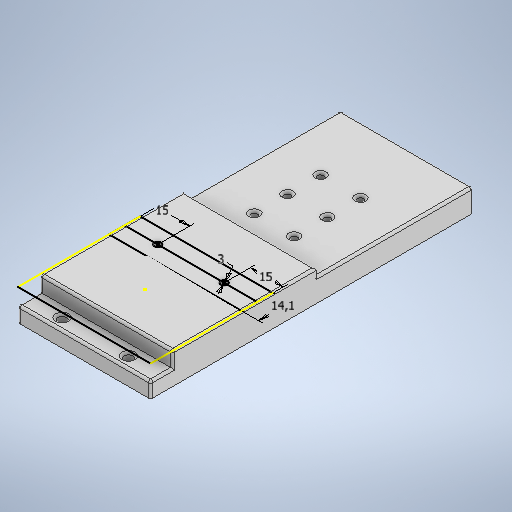
# Autodesk Inventor part: cadre
Saved by Autodesk Inventor 2025.1 (Build 291241000, 241)
## iProperties
Created: 2025-05-14
Part Number: cadre
Material: Générique
Document SubType Name: Modeling
Designer: chapuzet
Density: 1 g/cm^3
Appearance: Par défaut
Author: chapuzet
Autodesk Inventor part; units mm, degrees
ref_plane "YZ Plane" through (0, 0, 0) normal (1, 0, 0) x (0, 1, 0)
ref_plane "XZ Plane" through (0, 0, 0) normal (0, 1, 0) x (-1, 0, 0)
ref_plane "XY Plane" through (0, 0, 0) normal (0, 0, 1) x (1, 0, 0)
sketch "Esquisse1" plane through (0, 0, 0) normal (0, 1, 0) x (-1, 0, 0)
  line L0 (-30, 27.65) -> (30, 27.65)
  line L1 (30, 27.65) -> (30, -27.65)
  line L2 (30, -27.65) -> (-30, -27.65)
  line L3 (-30, -27.65) -> (-30, 27.65)
  line L4 (-30, 27.65) -> (30, -27.65) construction
  line L5 (30, 27.65) -> (-30, -27.65) construction
  point P0 (0, 0)
  dimension "d0" = 60
  dimension "d10" = 55.3
  constraints: 12 end point, 2 midpoint, 2 parallel, 1 horizontal, 1 perpendicular
  measures "d0" distance of L1.end L2.end
  measures "d10" distance of L0.end L1.end
extrude "Extrusion1" add sketch "Esquisse1" along normal blind 14
sketch "Esquisse2" plane through (0, 14, 0) normal (0, 1, 0) x (1, 0, 0)
  line L0 (30, -27.65) -> (30, 27.65) projected
  line L1 (-30, -27.65) -> (30, -27.65)
  line L2 (-30, 27.65) -> (-30, -27.65) projected
  line L3 (-30, 27.65) -> (30, 27.65)
  line L4 (30, 27.65) -> (30, 13.55)
  line L5 (30, 13.55) -> (-30, 13.55)
  line L6 (-30, 13.55) -> (-30, 27.65)
  line L7 (-30, 20.6) -> (30, 20.6)
  circle A0 centre (-15, 20.6) radius 1.5
  circle A1 centre (15, 20.6) radius 1.5
  point P0 (0, 0)
  point P1 (-30, 13.55)
  dimension "d29" = 14.1
  dimension "d40" = 15
  dimension "d41" = 15
  dimension "d42" = 3
  constraints: 12 end point, 3 point on line, 2 centre point, 2 horizontal, 2 midpoint, 2 parallel, 1 equal radius, 1 perpendicular
  measures "d29" distance between parallel lines of L3 L5
  measures "d40" distance from line of L0 A1.centre
  measures "d41" distance from line of L2 A0.centre
  measures "d42" diameter of A1
extrude "Extrusion2" [suppressed]
sketch "Esquisse5" plane through (30, 0, -27.65) normal (0, 0, -1) x (-1, 0, 0)
  line L0 (60, 0) -> (0, 0)
  line L1 (0, 0) -> (0, 14)
  line L2 (0, 14) -> (60, 14)
  line L3 (60, 14) -> (60, 0)
  point P0 (30, 0)
  constraints: 8 end point, 2 parallel, 1 horizontal, 1 perpendicular
extrude "Extrusion4" add sketch "Esquisse5" along normal blind 19.6
sketch "Esquisse6" plane through (30, 0, -47.25) normal (0, 0, -1) x (-1, 0, 0)
  line L0 (0, 0) -> (60, 0) projected
  line L1 (0, 14) -> (0, 0) projected
  line L2 (60, 0) -> (0, 0)
  line L3 (0, 0) -> (0, 10.4)
  line L4 (0, 10.4) -> (60, 10.4)
  line L5 (60, 10.4) -> (60, 0)
  point P0 (30, 0)
  point P1 (0, 15)
  dimension "d17" = 10.4
  constraints: 8 end point, 2 parallel, 1 horizontal, 1 perpendicular, 1 point on line
  measures "d17" distance between parallel lines of L0 L4
extrude "Extrusion5" add sketch "Esquisse6" along normal blind 71
sketch "Esquisse7" plane through (-30, 10.4, -47.25) normal (0, 1, 0) x (1, 0, 0)
  line L0 (0, -74.9) -> (0, 0) projected
  line L1 (0, 71) -> (60, 71) projected
  line L2 (0, 0) -> (60, 0)
  line L3 (60, 0) -> (60, 71)
  line L4 (60, 71) -> (0, 71)
  line L5 (0, 71) -> (0, 0)
  line L6 (21, 11) -> (39, 11)
  line L7 (39, 11) -> (39, 41)
  line L8 (39, 41) -> (21, 41)
  line L9 (21, 41) -> (21, 11)
  line L10 (21, 11) -> (39, 41) construction
  line L11 (39, 11) -> (21, 41) construction
  line L12 (30, 71) -> (30, 0)
  line L13 (39, 26) -> (21, 26)
  circle A0 centre (39, 11) radius 1.5
  circle A1 centre (21, 11) radius 1.5
  circle A2 centre (21, 26) radius 1.5
  circle A3 centre (39, 26) radius 1.5
  circle A4 centre (39, 41) radius 1.5
  circle A5 centre (21, 41) radius 1.5
  point P0 (30, -47.25)
  point P1 (0, -19.6)
  point P2 (30, 26)
  dimension "d20" = 18
  dimension "d21" = 11
  dimension "d22" = 30
  dimension "d23" = 3
  constraints: 24 end point, 6 centre point, 6 coincident, 6 midpoint, 5 equal radius, 4 parallel, 2 horizontal, 2 perpendicular, 1 point on line
  measures "d20" distance of L7.end L8.end
  measures "d21" distance between parallel lines of L2 L6
  measures "d22" distance of L6.end L7.end
  measures "d23" diameter of A0
extrude "Extrusion6" cut sketch "Esquisse7" against normal through all contours A4 L7 L8 | L8 L7 A4 | A5 L9 L8 | L8 L9 A5 | A3 L7 L13 | L13 L7 A3 | A2 L9 L13 | L13 L9 A2 | A1 L9 L6 | L6 L9 A1 | A0 L7 L6 | L6 L7 A0 | A3 L7 | L9 A2
sketch "Esquisse9" plane through (0, 14, 0) normal (0, 1, 0) x (1, 0, 0)
  line L0 (-30, -27.65) -> (30, -27.65) projected
  line L1 (-30, -27.65) -> (-30, 118.25) projected
  line L2 (30, -27.65) -> (-30, -27.65)
  line L3 (-30, -27.65) -> (-30, -17.65)
  line L4 (-30, -17.65) -> (30, -17.65)
  line L5 (30, -17.65) -> (30, -27.65)
  point P0 (0, 0)
  dimension "d30" = 10
  constraints: 8 end point, 2 parallel, 1 horizontal, 1 perpendicular, 1 point on line
  measures "d30" distance between parallel lines of L0 L4
extrude "Extrusion8" cut sketch "Esquisse9" against normal blind 7
sketch "Esquisse10" plane through (0, 7, 0) normal (0, 1, 0) x (1, 0, 0)
  line L0 (-30, -27.65) -> (-30, -17.65) projected
  line L1 (-30, -17.65) -> (30, -17.65) projected
  line L2 (-30, -27.65) -> (30, -27.65)
  line L3 (30, -27.65) -> (30, -17.65)
  line L4 (30, -17.65) -> (-30, -17.65)
  line L5 (-30, -17.65) -> (-30, -27.65)
  line L6 (-30, -22.65) -> (30, -22.65)
  circle A0 centre (15, -22.65) radius 2
  circle A1 centre (-15, -22.65) radius 2
  line L7 (30, -17.65) -> (30, -27.65) projected
  point P0 (0, 0)
  point P1 (0, -22.65)
  point P2 (-30, -22.65)
  dimension "d33" = 30
  dimension "d34" = 15
  dimension "d35" = 15
  dimension "d36" = 4
  constraints: 10 end point, 5 midpoint, 2 centre point, 2 parallel, 2 point on line, 1 equal radius, 1 horizontal, 1 perpendicular
  measures "d33" distance of point (30, -22.65) point (0, -22.65)
  measures "d34" distance from line of L7 A0.centre
  measures "d35" distance of A1.centre point (-30, -22.65)
  measures "d36" diameter of A0
extrude "Extrusion9" cut sketch "Esquisse10" against normal through all contours A1 L6 | L6 A1 | A0 L6 | L6 A0
fillet "Congé1" radius 1 30 edges at (0, 14, 17.65) (0, 7, 27.65) (30, 14, -14.8) (-30, 14, -14.8) (-30, 10.4, -82.75) (0, 10.4, -118.25) (-30, 5.2, -118.25) (-30, 3.5, 27.65) (30, 7, 22.65) (-30, 7, 22.65) (30, 3.5, 27.65) (30, 10.5, 17.65) (-30, 10.5, 17.65) (30, 10.4, -82.75) (30, 5.2, -118.25) (0, 14, -47.25) (7.5, 10.4, -58.25) (-10.5, 10.4, -58.25) (-10.5, 10.4, -73.25) (7.5, 10.4, -73.25) (7.5, 10.4, -88.25) (-10.5, 10.4, -88.25) (13, 7, 22.65) (-17, 7, 22.65) (7.5, 0, -58.25) (7.5, 0, -73.25) (7.5, 0, -88.25) (-10.5, 0, -88.25) (-10.5, 0, -73.25) (-10.5, 0, -58.25)
extrude "Extrusion10" cut sketch "Esquisse2" against normal through all contours A1 L7 | L7 A1 | A0 L7 | L7 A0
